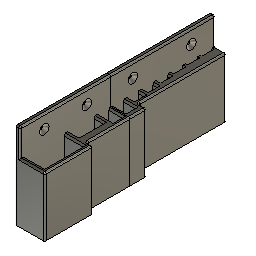
model (Autodesk Fusion 360 design; units mm, degrees)
Autodesk Fusion 360 part; units mm, degrees
note: some values were not read from the file. Set by a fixed rule: which sketch regions a step uses.
sketch "Sketch1" plane through (0, 0, 0) normal (0, 0, 1) x (1, 0, 0)
  line L0 (228.1, 6.3) -> (241.6, 6.3)
  line L1 (241.6, 6.3) -> (241.6, 5)
  line L2 (241.6, 5) -> (228.1, 5)
  line L3 (228.1, 5) -> (228.1, 6.3)
  line L4 (0, 5) -> (241.5893, 5)
  line L5 (209.6, 5) -> (223.1, 5)
  line L6 (223.1, 5) -> (223.1, 6.8)
  line L7 (223.1, 6.8) -> (209.6, 6.8)
  line L8 (209.6, 6.8) -> (209.6, 5)
  line L9 (228.1, 5.65) -> (223.1, 5.65) construction
  line L10 (191.1, 5) -> (204.6, 5)
  line L11 (204.6, 5) -> (204.6, 7.8)
  line L12 (204.6, 7.8) -> (191.1, 7.8)
  line L13 (191.1, 7.8) -> (191.1, 5)
  line L14 (209.6, 5.9) -> (204.6, 5.9) construction
  line L15 (186.1, 5) -> (172.6, 5)
  line L16 (172.6, 5) -> (172.6, 9.8)
  line L17 (172.6, 9.8) -> (186.1, 9.8)
  line L18 (186.1, 9.8) -> (186.1, 5)
  line L19 (167.6, 5) -> (154.1, 5)
  line L20 (154.1, 5) -> (154.1, 12.3)
  line L21 (154.1, 12.3) -> (167.6, 12.3)
  line L22 (167.6, 12.3) -> (167.6, 5)
  line L23 (149.1, 5) -> (135.6, 5)
  line L24 (135.6, 5) -> (135.6, 13.8)
  line L25 (135.6, 13.8) -> (149.1, 13.8)
  line L26 (149.1, 13.8) -> (149.1, 5)
  line L27 (130.6, 5) -> (117.1, 5)
  line L28 (117.1, 5) -> (117.1, 21.8)
  line L29 (117.1, 21.8) -> (130.6, 21.8)
  line L30 (130.6, 21.8) -> (130.6, 5)
  line L31 (112.1, 5) -> (98.6, 5)
  line L32 (98.6, 5) -> (98.6, 23.8)
  line L33 (98.6, 23.8) -> (112.1, 23.8)
  line L34 (112.1, 23.8) -> (112.1, 5)
  line L35 (93.6, 5) -> (60.8, 5)
  line L36 (60.8, 5) -> (60.8, 18.5)
  line L37 (60.8, 18.5) -> (93.6, 18.5)
  line L38 (93.6, 18.5) -> (93.6, 5)
  line L39 (55.8, 5) -> (5, 5)
  line L40 (5, 5) -> (5, 30.8)
  line L41 (5, 30.8) -> (55.8, 30.8)
  line L42 (55.8, 30.8) -> (55.8, 5)
  line L43 (191.1, 6.4) -> (186.1, 6.4) construction
  line L44 (172.6, 7.4) -> (167.6, 7.4) construction
  line L45 (154.1, 8.65) -> (149.1, 8.65) construction
  line L46 (135.6, 9.4) -> (130.6, 9.4) construction
  line L47 (117.1, 13.4) -> (112.1, 13.4) construction
  line L48 (98.6, 14.4) -> (93.6, 14.4) construction
  line L49 (60.8, 11.75) -> (55.8, 11.75) construction
  line L50 (5, 17.9) -> (0, 17.9) construction
  line L51 (241.6, 5.65) -> (246.6, 5.65) construction
  line L52 (5, 5) -> (5, 0) construction
  line L53 (184.5, 6.6) -> (174.2, 6.6)
  line L54 (174.2, 6.6) -> (174.2, 8.2)
  line L55 (174.2, 8.2) -> (184.5, 8.2)
  line L56 (184.5, 8.2) -> (184.5, 6.6)
  line L57 (155.7, 6.6) -> (155.7, 10.7)
  line L58 (155.7, 10.7) -> (166, 10.7)
  line L59 (166, 10.7) -> (166, 6.6)
  line L60 (166, 6.6) -> (155.7, 6.6)
  line L61 (137.2, 6.6) -> (137.2, 12.2)
  line L62 (137.2, 12.2) -> (147.5, 12.2)
  line L63 (147.5, 12.2) -> (147.5, 6.6)
  line L64 (147.5, 6.6) -> (137.2, 6.6)
  line L65 (118.7, 6.6) -> (118.7, 20.2)
  line L66 (118.7, 20.2) -> (129, 20.2)
  line L67 (129, 20.2) -> (129, 6.6)
  line L68 (129, 6.6) -> (118.7, 6.6)
  line L69 (100.2, 6.6) -> (100.2, 22.2)
  line L70 (100.2, 22.2) -> (110.5, 22.2)
  line L71 (110.5, 22.2) -> (110.5, 6.6)
  line L72 (110.5, 6.6) -> (100.2, 6.6)
  line L73 (62.4, 6.6) -> (62.4, 16.9)
  line L74 (62.4, 16.9) -> (92, 16.9)
  line L75 (92, 16.9) -> (92, 6.6)
  line L76 (92, 6.6) -> (62.4, 6.6)
  line L77 (6.6, 6.6) -> (6.6, 29.2)
  line L78 (6.6, 29.2) -> (54.2, 29.2)
  line L79 (54.2, 29.2) -> (54.2, 6.6)
  line L80 (54.2, 6.6) -> (6.6, 6.6)
  line L81 (221.5, 5) -> (221.5, 6.8)
  line L82 (211.2, 5) -> (211.2, 6.8)
  line L83 (240, 5) -> (240, 6.3)
  line L84 (229.7, 5) -> (229.7, 6.3)
  line L85 (246.6, 0) -> (0, 0)
  line L86 (203, 5) -> (203, 7.8)
  line L87 (192.7, 5) -> (192.7, 7.8)
  line L88 (0, 0) -> (0, 35.8)
  line L89 (246.6, 0) -> (246.6, 18.8)
  line L90 (0, 35.8) -> (60.8, 35.8)
  line L91 (60.8, 35.8) -> (60.8, 28.8)
  line L92 (60.8, 28.8) -> (135.6, 28.8)
  line L93 (135.6, 28.8) -> (135.6, 18.8)
  line L94 (135.6, 18.8) -> (246.6, 18.8)
  line L95 (30.4, 30.8) -> (30.4, 35.8) construction
  line L96 (105.35, 23.8) -> (105.35, 28.8) construction
  line L97 (142.35, 13.8) -> (142.35, 18.8) construction
  line L98 (135.6, 18.8) -> (130.6, 18.8) construction
  line L99 (60.8, 28.8) -> (55.8, 28.8) construction
  line L100 (241.5893, 5) -> (246.6, 5)
  dimension "d4" = 13.5
  dimension "d5" = 1.3
  dimension "d6" = 1.8
  dimension "d7" = 5
  dimension "d8" = 2.8
  dimension "d9" = 4.8
  dimension "d10" = 7.3
  dimension "d11" = 8.8
  dimension "d12" = 16.8
  dimension "d13" = 18.8
  dimension "d14" = 32.8
  dimension "d15" = 25.8
  dimension "d16" = 50.8
  dimension "d24" = 1.6
  dimension "d25" = 1.6
  dimension "d26" = 1.6
  dimension "d27" = 1.6
  dimension "d28" = 1.6
  dimension "d29" = 1.6
  dimension "d30" = 1.6
  dimension "d31" = 1.6
  dimension "d32" = 1.6
  dimension "d33" = 1.6
  dimension "d34" = 1.6
  dimension "d63" = 1.6
  dimension "d64" = 1.6
  constraint horizontal L0
  constraint vertical L1
  constraint horizontal L2
  constraint vertical L3
  constraint coincident L1.end L4
  constraint horizontal L5
  constraint vertical L6
  constraint horizontal L7
  constraint vertical L8
  constraint coincident L4 L5.start
  constraint equal L0 L7
  constraint midpoint L3 L9.start
  constraint coincident L6 L9.end
  constraint horizontal L9
  constraint horizontal L4
  constraint horizontal L10
  constraint vertical L11
  constraint horizontal L12
  constraint vertical L13
  constraint coincident L4 L10.start
  constraint equal L7 L12
  constraint midpoint L8 L14.start
  constraint coincident L11 L14.end
  constraint perpendicular L11 L14
  constraint equal L9 L14
  constraint horizontal L15
  constraint vertical L16
  constraint horizontal L17
  constraint vertical L18
  constraint coincident L4 L15.start
  constraint horizontal L19
  constraint vertical L20
  constraint horizontal L21
  constraint vertical L22
  constraint coincident L4 L19.start
  constraint horizontal L23
  constraint vertical L24
  constraint horizontal L25
  constraint vertical L26
  constraint coincident L4 L23.start
  constraint horizontal L27
  constraint vertical L28
  constraint horizontal L29
  constraint vertical L30
  constraint coincident L4 L27.start
  constraint horizontal L31
  constraint vertical L32
  constraint horizontal L33
  constraint vertical L34
  constraint coincident L4 L31.start
  constraint horizontal L35
  constraint vertical L36
  constraint horizontal L37
  constraint vertical L38
  constraint coincident L4 L35.start
  constraint horizontal L39
  constraint vertical L40
  constraint horizontal L41
  constraint vertical L42
  constraint coincident L4 L39.start
  constraint midpoint L13 L43.start
  constraint coincident L18 L43.end
  constraint perpendicular L18 L43
  constraint midpoint L16 L44.start
  constraint coincident L22 L44.end
  constraint perpendicular L22 L44
  constraint midpoint L20 L45.start
  constraint coincident L26 L45.end
  constraint perpendicular L26 L45
  constraint midpoint L24 L46.start
  constraint coincident L30 L46.end
  constraint perpendicular L30 L46
  constraint midpoint L28 L47.start
  constraint coincident L34 L47.end
  constraint perpendicular L34 L47
  constraint midpoint L32 L48.start
  constraint coincident L38 L48.end
  constraint perpendicular L38 L48
  constraint midpoint L36 L49.start
  constraint coincident L42 L49.end
  constraint perpendicular L42 L49
  constraint equal L14 L43
  constraint equal L43 L44
  constraint equal L44 L45
  constraint equal L45 L46
  constraint equal L46 L47
  constraint equal L47 L48
  constraint equal L48 L49
  constraint equal L12 L17
  constraint equal L17 L21
  constraint equal L21 L25
  constraint equal L25 L29
  constraint equal L29 L33
  constraint equal L33 L38
  constraint midpoint L40 L50.start
  constraint midpoint L1 L51.start
  constraint equal L9 L51
  constraint equal L50 L51
  constraint equal L50 L52
  constraint coincident L5 L81.start
  constraint coincident L7 L81.end
  constraint perpendicular L7 L81
  constraint coincident L5 L82.start
  constraint coincident L7 L82.end
  constraint perpendicular L7 L82
  constraint coincident L2 L83.start
  constraint coincident L0 L83.end
  constraint perpendicular L0 L83
  constraint coincident L2 L84.start
  constraint coincident L0 L84.end
  constraint perpendicular L0 L84
  constraint coincident L85.end L88.start
  constraint coincident L52.end L85
  constraint horizontal L85
  constraint vertical L52
  constraint horizontal L51
  constraint horizontal L50
  constraint coincident L10 L86.start
  constraint coincident L12 L86.end
  constraint perpendicular L12 L86
  constraint coincident L10 L87.start
  constraint coincident L12 L87.end
  constraint perpendicular L12 L87
  constraint perpendicular L85 L88
  constraint coincident L50.end L88
  constraint perpendicular L85 L89
  constraint coincident L51.end L89
  constraint horizontal L94
  constraint vertical L93
  constraint horizontal L92
  constraint vertical L91
  constraint horizontal L90
  constraint midpoint L41 L95.start
  constraint coincident L90 L95.end
  constraint perpendicular L90 L95
  constraint midpoint L33 L96.start
  constraint coincident L92 L96.end
  constraint perpendicular L92 L96
  constraint midpoint L25 L97.start
  constraint coincident L94 L97.end
  constraint perpendicular L94 L97
  constraint coincident L30 L98.end
  constraint horizontal L98
  constraint equal L51 L97
  constraint equal L97 L98
  constraint equal L96 L98
  constraint equal L95 L96
  constraint coincident L42 L99.end
  constraint perpendicular L42 L99
  constraint equal L95 L99
  constraint coincident L89 L100.end
  constraint perpendicular L89 L100
  constraint coincident L4.start L88
  measures "d4" distance of L1.end L2.end
  measures "d5" distance of L0.end L1.end
  measures "d6" distance of L5.end L6.end
  measures "d7" distance of L9.start L9.end
  measures "d8" distance of L10.end L11.end
  measures "d9" distance of L15.start L17.end
  measures "d10" distance of L19.start L21.end
  measures "d11" distance of L23.start L25.end
  measures "d12" distance of L27.start L29.end
  measures "d13" distance of L31.start L33.end
  measures "d14" distance of L35.start L35.end
  measures "d15" distance of L39.end L40.end
  measures "d16" distance of L39.start L39.end
  measures "d31" distance of L1.end L83.start
  measures "d32" distance of L2.end L84.start
  measures "d33" distance of L5.end L81.start
  measures "d34" distance of L5.start L82.start
  measures "d63" distance of L10.end L86.start
  measures "d64" distance of L10.start L87.start
extrude "Extrude1" add sketch "Sketch1" along normal blind 111.65 contours L2 L4 L5 L10 L15 L19 L23 L27 L31 L35 L39 L85 L88 L89 L100 makes body 1
extrude "Extrude2" add sketch "Sketch1" along normal blind 77.14 contours L0 L1 L3 L4 L6 L7 L8 L11 L12 L13 L16 L17 L18 L20 L21 L22 L24 L25 L26 L28 L29 L30 L32 L33 L34 L36 L37 L38 L40 L41 L42 L88 L89 L90 L91 L92 L93 L94 L100 bodies 1
sketch "Sketch2" plane through (0, 5, 0) normal (0, 1, 0) x (-1, 0, 0)
  line L0 (-241.6, 77.14) -> (-241.6, 0)
  line L1 (-204.6, 0) -> (-191.1, 0)
  line L2 (0, 111.65) -> (-246.6, 111.65)
  line L3 (-246.6, 94.395) -> (0, 94.395) construction
  circle A0 centre (-216.35, 94.395) radius 2
  circle A1 centre (-30.4, 94.395) radius 2
  line L4 (-114.6, 77.14) -> (-114.6, 94.395) construction
  circle A2 centre (-142.35, 94.395) radius 2
  line L5 (-216.35, 0) -> (-216.35, 94.395) construction
  line L6 (-142.35, 94.395) -> (-142.35, 0) construction
  line L7 (-30.4, 94.395) -> (-30.4, 0) construction
  circle A3 centre (-84.2, 94.395) radius 2
  line L8 (-98.6, 0) -> (-98.6, 77.14)
  line L9 (-112.1, 77.14) -> (-112.1, 0)
  line L10 (-135.6, 0) -> (-135.6, 77.14)
  line L11 (-149.1, 77.14) -> (-149.1, 0)
  line L12 (-60.8, 0) -> (-60.8, 77.14)
  line L13 (-93.6, 77.14) -> (-93.6, 0)
  line L14 (-117.1, 0) -> (-117.1, 77.14)
  line L15 (-130.6, 77.14) -> (-130.6, 0)
  line L16 (-172.6, 0) -> (-172.6, 77.14)
  line L17 (-186.1, 77.14) -> (-186.1, 0)
  line L18 (-5, 0) -> (-5, 77.14)
  line L19 (-55.8, 77.14) -> (-55.8, 0)
  line L20 (-209.6, 0) -> (-209.6, 77.14)
  line L21 (-223.1, 77.14) -> (-223.1, 0)
  line L22 (-191.1, 0) -> (-191.1, 77.14)
  line L23 (-204.6, 77.14) -> (-204.6, 0)
  line L24 (-154.1, 0) -> (-154.1, 77.14)
  line L25 (-167.6, 77.14) -> (-167.6, 0)
  line L26 (-209.6, 77.14) -> (-204.6, 77.14)
  line L27 (-191.1, 77.14) -> (-186.1, 77.14)
  line L28 (-186.1, 0) -> (-172.6, 0)
  line L29 (-172.6, 77.14) -> (-167.6, 77.14)
  line L30 (-167.6, 0) -> (-154.1, 0)
  line L31 (-154.1, 77.14) -> (-149.1, 77.14)
  line L32 (-149.1, 0) -> (-135.6, 0)
  line L33 (-135.6, 77.14) -> (-130.6, 77.14)
  line L34 (-130.6, 0) -> (-117.1, 0)
  line L35 (-117.1, 77.14) -> (-112.1, 77.14)
  line L36 (-112.1, 0) -> (-98.6, 0)
  line L37 (-98.6, 77.14) -> (-93.6, 77.14)
  line L38 (-93.6, 0) -> (-60.8, 0)
  line L39 (-60.8, 77.14) -> (-55.8, 77.14)
  line L40 (-55.8, 0) -> (-5, 0)
  line L41 (-5, 77.14) -> (0, 77.14)
  line L42 (0, 77.14) -> (0, 111.65)
  line L43 (-246.6, 111.65) -> (-246.6, 77.14)
  line L44 (-246.6, 77.14) -> (-241.6, 77.14)
  line L45 (-241.6, 0) -> (-228.1, 0)
  line L46 (-228.1, 0) -> (-228.1, 77.14)
  line L47 (-228.1, 77.14) -> (-223.1, 77.14)
  line L48 (-223.1, 0) -> (-209.6, 0)
  dimension "d55" = 4
  dimension "d60" = 30.4
  dimension "d61" = 30.4
  constraint coincident L3 A0.centre
  constraint coincident L3 A1.centre
  constraint equal A0 A1
  constraint coincident L3 L4.end
  constraint perpendicular L3 L4
  constraint coincident L3 A2.centre
  constraint equal A0 A2
  constraint coincident A0.centre L5.end
  constraint vertical L5
  constraint coincident A2.centre L6.start
  constraint vertical L6
  constraint coincident A1.centre L7.start
  constraint vertical L7
  constraint coincident L3 A3.centre
  constraint equal A1 A3
  constraint midpoint L3.start L43
  constraint midpoint L3.end L42
  constraint midpoint L6.end L32
  constraint midpoint L5.start L48
  constraint midpoint L4.start L35
  constraint midpoint L7.end L40
  measures "d55" diameter of A0
  measures "d60" distance of L4.end A3.centre
  measures "d61" distance of L3.end A1.centre
extrude "Extrude3" add sketch "Sketch1" along normal blind 2 contours L0 L2 L3 L4 L84 | L0 L1 L2 L4 L83 L100 | L4 L5 L6 L7 L81 | L4 L5 L7 L8 L82 | L4 L10 L11 L12 L86 | L4 L10 L12 L13 L87 | L4 L15 L16 L17 L18 | L4 L35 L36 L37 L38 | L4 L19 L20 L21 L22 | L4 L31 L32 L33 L34 | L4 L23 L24 L25 L26 | L4 L27 L28 L29 L30 bodies 1
extrude "Extrude4" add sketch "Sketch1" along normal up to surface (3.5 mm away) contours L4 L39 L40 L41 L42 bodies 1
chamfer "Chamfer1" distance 1 distance2 3 20 edges at (241.6, 5.65, 77.14) (228.1, 5.65, 77.14) (223.1, 5.9, 77.14) (209.6, 5.9, 77.14) (204.6, 6.4, 77.14) (191.1, 6.4, 77.14) (186.1, 7.4, 77.14) (172.6, 7.4, 77.14) (167.6, 8.65, 77.14) (154.1, 8.65, 77.14) (149.1, 9.4, 77.14) (135.6, 9.4, 77.14) (130.6, 13.4, 77.14) (117.1, 13.4, 77.14) (112.1, 14.4, 77.14) (98.6, 14.4, 77.14) (93.6, 11.75, 77.14) (60.8, 11.75, 77.14) (55.8, 17.9, 77.14) (5, 17.9, 77.14) measured on face at (71.7333, 21.9333, 77.14) measured on face at (71.7333, 21.9333, 77.14) measured on face at (71.7333, 21.9333, 77.14) measured on face at (71.7333, 21.9333, 77.14) measured on face at (71.7333, 21.9333, 77.14) measured on face at (71.7333, 21.9333, 77.14) measured on face at (71.7333, 21.9333, 77.14) measured on face at (71.7333, 21.9333, 77.14) measured on face at (71.7333, 21.9333, 77.14) measured on face at (71.7333, 21.9333, 77.14) measured on face at (71.7333, 21.9333, 77.14) measured on face at (71.7333, 21.9333, 77.14) measured on face at (71.7333, 21.9333, 77.14) measured on face at (71.7333, 21.9333, 77.14) measured on face at (71.7333, 21.9333, 77.14) measured on face at (71.7333, 21.9333, 77.14) measured on face at (71.7333, 21.9333, 77.14) measured on face at (71.7333, 21.9333, 77.14) measured on face at (71.7333, 21.9333, 77.14) measured on face at (71.7333, 21.9333, 77.14) on bodies 1
chamfer "Chamfer2" distance 1 angle 45 10 edges at (234.85, 6.3, 77.14) (216.35, 6.8, 77.14) (197.85, 7.8, 77.14) (179.35, 9.8, 77.14) (160.85, 12.3, 77.14) (142.35, 13.8, 77.14) (123.85, 21.8, 77.14) (105.35, 23.8, 77.14) (77.2, 18.5, 77.14) (30.4, 30.8, 77.14) on bodies 1
extrude "Extrude6" cut sketch "Sketch2" against normal up to surface (5 mm away) contours A0 | A1 | A2 | A3 bodies 1
chamfer "Chamfer4" distance 4 angle 45 4 edges at (218.2147, 5, 95.1182) (144.2147, 5, 95.1182) (86.0647, 5, 95.1182) (32.2647, 5, 95.1182) on bodies 1
ref_plane "WorkPlane1" through (114.6, 5, 85.7675) normal (-1, 0, 0) x (0, 0, 1)
split "Split1" by plane through (114.6, 5, 85.7675) normal (-1, 0, 0) bodies 1 makes body 2 at (48.636, 0, 30.871)
fillet "Fillet4" radius 2 20 edges at (246.6, 2.5, 111.65) (246.6, 18.8, 38.57) (135.6, 28.8, 38.57) (135.6, 18.8, 38.57) (180.6, 5, 111.65) (246.6, 5, 94.395) (246.6, 11.9, 77.14) (191.1, 18.8, 77.14) (135.6, 23.8, 77.14) (125.1, 28.8, 77.14) (0, 2.5, 111.65) (60.8, 35.8, 38.57) (0, 35.8, 38.57) (0, 5, 94.395) (57.3, 5, 111.65) (87.7, 28.8, 77.14) (60.8, 32.3, 77.14) (30.4, 35.8, 77.14) (0, 20.4, 77.14) (60.8, 28.8, 38.57) on bodies 1 2
chamfer "Chamfer5" distance 2 angle 45 14 edges at (88.7, 28.8, 0) (0, 16.9, 0) (0.5858, 35.2142, 0) (30.4, 35.8, 0) (60.2142, 35.2142, 0) (60.8, 32.3, 0) (61.3858, 29.3858, 0) (191.1, 18.8, 0) (246.0142, 18.2142, 0) (246.6, 8.4, 0) (124.1, 28.8, 0) (135.0142, 28.2142, 0) (135.6, 23.8, 0) (136.1858, 19.3858, 0) on bodies 1 2
mirror "Mirror1" about plane through (114.6, 5, 85.7675) normal (-1, 0, 0) of bodies 1 2 makes body 3 at (37.6994, 0, 30.8973) makes body 4 at (162.5693, 0, 30.871)
hidden bodies 1 2
equation "margin = 0.8 mm"
equation "clearance = 5 mm"
equation "width = 12.7 mm"
equation "d4 = width + margin"
equation "d5 = 0.5 mm + margin"
equation "d6 = 1 mm + margin"
equation "d7 = clearance"
equation "d8 = 2 mm + margin"
equation "d9 = 4 mm + margin"
equation "d10 = 6.5 mm + margin"
equation "d11 = 8 mm + margin"
equation "d12 = 16 mm + margin"
equation "d13 = 18 mm + margin"
equation "d14 = 32 mm + margin"
equation "d15 = 25 mm + margin"
equation "d16 = 50 mm + margin"
equation "height = 101.5 mm"
equation "d20 = height * 1.1"
equation "lip = 2 * margin"
equation "d24 = lip"
equation "d25 = lip"
equation "d26 = lip"
equation "d27 = lip"
equation "d28 = lip"
equation "d29 = lip"
equation "d30 = lip"
equation "d31 = lip"
equation "d32 = lip"
equation "d33 = lip"
equation "d34 = lip"
equation "d36 = height * 0.76"
equation "d60 = d61"
equation "d63 = lip"
equation "d64 = lip"
